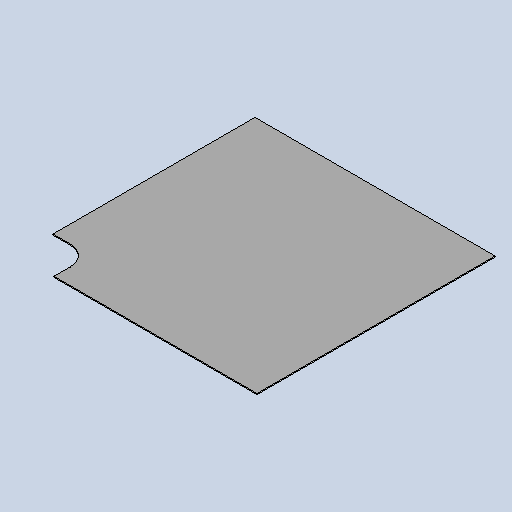
# Autodesk Inventor part: PNS waste water bin 07
Saved by Autodesk Inventor 2025.3 (Build 293356030, 356C)
## iProperties
Created: 2025-09-03
Part Number: PNS waste water bin 07
Material: Generic
Document SubType Name: Sheet Metal
Designer: admin
Density: 1 g/cm^3
Sheet Metal Rule: Default
Appearance: Default
Flat Pattern Width: 47.5 cm
Flat Pattern Length: 47.9 cm
Flat Pattern Area: 2275.25 cm^2
Sheet Metal Width: 475,000 mm
Sheet Metal Length: 479,000 mm
Sheet Metal Area: 227525,000 mm^2
Mass: 445.081 g
Surface Area: 4488.62 cm^2
Volume: 445.081 cm^3
Author: admin
Autodesk Inventor part; units mm, degrees
ref_plane "YZ Plane" through (0, 0, 0) normal (1, 0, 0) x (0, 1, 0)
ref_plane "XZ Plane" through (0, 0, 0) normal (0, 1, 0) x (-1, 0, 0)
ref_plane "XY Plane" through (0, 0, 0) normal (0, 0, 1) x (1, 0, 0)
sketch "Sketch1" plane through (0, 0, 0) normal (0, 0, 1) x (1, 0, 0)
  line L0 (239.5, 237.5) -> (-239.5, -237.5) construction
  line L1 (-239.5, -237.5) -> (239.5, -237.5)
  line L2 (239.5, -237.5) -> (239.5, 237.5)
  line L3 (239.5, 237.5) -> (-239.5, 237.5)
  line L4 (-239.5, 237.5) -> (-239.5, -237.5)
  line L5 (-239.5, -237.5) -> (239.5, 237.5) construction
  line L6 (239.5, -237.5) -> (-239.5, 237.5) construction
  line L7 (-165.5, -237.5) -> (-165.5, -205.5)
  arc A0 (-165.5, -205.5) -> (-205.5, -165.5) centre (-205.5, -205.5) ccw
  line L8 (-205.5, -165.5) -> (-239.5, -165.5)
  point P0 (0, 0)
  dimension "d2" = 479
  dimension "d18" = 475
  dimension "d21" = 40
  dimension "d22" = 72
  dimension "d23" = 74
  measures "d2" distance of L3.end L2.end
  measures "d18" distance of L1.end L2.end
  measures "d21" radius of A0
  measures "d22" distance between parallel lines of L1 L8
  measures "d23" distance between parallel lines of L4 L7
extrude "Plate1" add sketch "Sketch1" along normal blind 2 contours L7 A0 L8 L4 L3 L2 L1
equation "\"d3\" = Thickness"
equation "\"BendRadius\" = Thickness"
equation "\"BendReliefWidth\" = Thickness"
equation "\"BendReliefDepth\" = 0.5 * Thickness"
equation "\"CornerReliefSize\" = 4 * Thickness"
equation "\"MinimumRemnant\" = 2 * Thickness"
equation "\"TransitionRadius\" = BendRadius"
equation "\"JacobiRadiusSize\" = BendRadius"
equation "\"GapSize\" = Thickness"
equation "\"Thickness\" = 2"
body "Solid1"
